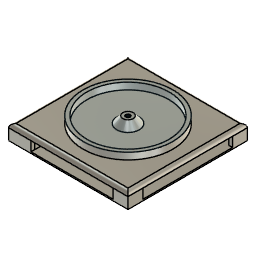
LED Box Holder (Autodesk Fusion 360 design; units mm, degrees)
Autodesk Fusion 360 part; units mm, degrees
sketch "Sketch1" plane through (0, 0, 0) normal (1, 0, 0) x (0, 1, 0)
  line L0 (-80, 80) -> (80, 80)
  line L1 (80, 80) -> (80, -80)
  line L2 (80, -80) -> (-80, -80)
  line L3 (-80, -80) -> (-80, 80)
  line L4 (-80, 80) -> (80, -80) construction
  line L5 (80, 80) -> (-80, -80) construction
  dimension "d1" = 160
  dimension "d2" = 160
  constraint horizontal L0
  constraint perpendicular L0 L1
  constraint parallel L0 L2
  constraint parallel L1 L3
  constraint coincident L4 origin
  constraint coincident L5 origin
  measures "d1" distance of L1.end L2.end
  measures "d2" distance of L0.end L1.end
extrude "Extrude1" add sketch "Sketch1" along normal blind 5 makes body 1
sketch "Sketch2" plane through (5, 0, 0) normal (1, 0, 0) x (0, 1, 0)
  line L0 (-80, -80) -> (80, -80)
  line L1 (80, -80) -> (80, 80)
  line L2 (80, 80) -> (-80, 80)
  line L3 (-80, 80) -> (-80, -80)
  line L4 (-55, 50) -> (55, 50)
  line L5 (55, 50) -> (55, 35)
  line L6 (55, 35) -> (-55, 35)
  line L7 (-55, 35) -> (-55, 50)
  dimension "d5" = 110
  dimension "d6" = 15
  dimension "d7" = 30
  dimension "d8" = 25
  constraint horizontal L4
  constraint vertical L5
  constraint horizontal L6
  constraint vertical L7
  measures "d5" distance of L4.start L4.end
  measures "d6" distance of L4.start L6.end
  measures "d7" distance of L2 L4
  measures "d8" distance of L1 L5
extrude "Extrude2" cut sketch "Sketch2" against normal blind 20 contours L4 L5 L6 L7 bodies 1
sketch "Sketch3" plane through (0, 0, 0) normal (-1, 0, 0) x (0, -1, 0)
  line L0 (-55, 35) -> (-55, 50)
  line L1 (-55, 50) -> (55, 50)
  line L2 (55, 50) -> (55, 35)
  line L3 (55, 35) -> (-55, 35)
  line L4 (-80, -80) -> (80, -80)
  line L5 (80, -80) -> (80, 80)
  line L6 (80, 80) -> (-80, 80)
  line L7 (-80, 80) -> (-80, -80)
  line L8 (-50, 35) -> (-30, 35)
  line L9 (-30, 35) -> (-30, -80)
  line L10 (-30, -80) -> (-50, -80)
  line L11 (-50, -80) -> (-50, 35)
  line L12 (-10, 35) -> (10, 35)
  line L13 (10, 35) -> (10, -80)
  line L14 (10, -80) -> (-10, -80)
  line L15 (-10, -80) -> (-10, 35)
  line L16 (30, 35) -> (50, 35)
  line L17 (50, 35) -> (50, -80)
  line L18 (50, -80) -> (30, -80)
  line L19 (30, -80) -> (30, 35)
  dimension "d11" = 20
  dimension "d12" = 115
  dimension "d13" = 20
  dimension "d14" = 115
  dimension "d15" = 5
  dimension "d17" = 20
  dimension "d18" = 20
  dimension "d19" = 115
  constraint horizontal L8
  constraint vertical L9
  constraint horizontal L10
  constraint vertical L11
  constraint coincident L3 L8.start
  constraint horizontal L12
  constraint vertical L13
  constraint horizontal L14
  constraint vertical L15
  constraint coincident L3 L12.start
  constraint horizontal L16
  constraint vertical L17
  constraint horizontal L18
  constraint vertical L19
  constraint coincident L3 L16.start
  measures "d11" distance of L8.start L8.end
  measures "d12" distance of L8.start L10.end
  measures "d13" distance of L12.start L12.end
  measures "d14" distance of L12.start L14.end
  measures "d15" distance of L0 L11
  measures "d17" distance of L9 L15
  measures "d18" distance of L13 L19
  measures "d19" distance of L16 L18
extrude "Extrude3" cut sketch "Sketch3" against normal blind 3 contours L3 L4 L8 L9 L10 L11 | L3 L4 L12 L13 L14 L15 | L3 L4 L16 L17 L18 L19 bodies 1
extrude "Extrude4" add 3 faces at (0, 18.3333, 70) (0, 23.3333, -41.6667) (0, -23.3333, -3.3333) along direction (-1, 0, 0) blind 10 on bodies 1 bodies 1
sketch "Sketch4" plane through (-10, 0, 0) normal (-1, 0, 0) x (0, -1, 0)
  line L0 (-50, -80) -> (-50, 35)
  line L1 (-50, 35) -> (-55, 35)
  line L2 (-55, 35) -> (-55, 50)
  line L3 (-55, 50) -> (55, 50)
  line L4 (55, 50) -> (55, 35)
  line L5 (55, 35) -> (50, 35)
  line L6 (50, 35) -> (50, -80)
  line L7 (50, -80) -> (80, -80)
  line L8 (80, -80) -> (80, 80)
  line L9 (80, 80) -> (-80, 80)
  line L10 (-80, 80) -> (-80, -80)
  line L11 (-80, -80) -> (-50, -80)
  line L12 (-80, -80) -> (80, -80)
  line L13 (80, -80) -> (80, 80)
  line L14 (80, 80) -> (-80, 80)
  line L15 (-80, 80) -> (-80, -80)
  dimension "d24" = 160
  constraint horizontal L12
  constraint vertical L13
  constraint horizontal L14
  constraint vertical L15
  constraint coincident L10.end L11.start
  measures "d24" distance of L10.end L9.end
extrude "Extrude5" add sketch "Sketch4" along normal blind 5 bodies 1
fillet "Fillet1" radius 5 4 edges at (-15, 0, 80) (-15, 80, 0) (-15, -80, 0) (-15, 0, -80) on bodies 1
sketch "Sketch5" plane through (-15, 0, 0) normal (-1, 0, 0) x (0, -1, 0)
  line L0 (-75, -75) -> (75, -75)
  line L1 (75, -75) -> (75, 75)
  line L2 (75, 75) -> (-75, 75)
  line L3 (-75, 75) -> (-75, -75)
  circle A0 centre (0, 0) radius 60
  constraint coincident A0.centre origin
extrude "Extrude6" add sketch "Sketch5" along normal blind 9 contours A0 bodies 1
sketch "Sketch6" plane through (-24, 0, 0) normal (-1, 0, 0) x (0, -1, 0)
  circle A0 centre (0, 0) radius 60
  circle A1 centre (0, 0) radius 3
  dimension "d31" = 6
  constraint coincident A0.centre A1.centre
  measures "d31" diameter of A1
extrude "Extrude7" cut sketch "Sketch6" against normal blind 10 contours A1 bodies 1
thread "Thread1" "ISO Metric profile 6.0 M6x1 6H" major diameter 6.147 minor diameter 5.035 pitch 1 angle 60 modelled right hand crest width 0.2748 on face at (-17.3333, -2.9963, -0.1495) crest through (-23.75, -2.5175, 0) on bodies 1
sketch "Sketch7" plane through (-24, 0, 0) normal (-1, 0, 0) x (0, -1, 0)
  spline S0 degree 3 poles (-0.7938, -2.9692) (-1.1619, -2.8346) (-1.5007, -2.6305) (-2.069, -2.1114) (-2.2965, -1.8052) (-2.6132, -1.1343) (-2.704, -0.7783) (-2.7408, -0.0652) (-2.6916, 0.2847) (-2.5067, 0.8107) (-2.4149, 0.9977) (-2.1912, 1.3413) (-2.061, 1.4974) (-1.9135, 1.636) knots 0 0 0 0 0.117588 0.117588 0.231087 0.231087 0.340498 0.340498 0.445817 0.445817 0.508297 0.508297 0.569249 0.569249 0.569249 0.569249
  arc A0 (1.9135, 1.636) -> (-1.9135, 1.636) centre (0, 0) ccw
  spline S1 degree 3 poles (1.9135, 1.636) (2.1558, 1.4082) (2.3504, 1.1345) (2.6319, 0.5162) (2.7113, 0.1755) (2.7381, -0.5311) (2.68, -0.8904) (2.4271, -1.5805) (2.2298, -1.9028) (1.817, -2.3542) (1.6364, -2.5092) (1.2382, -2.776) (1.0214, -2.886) (0.7938, -2.9692) knots 0 0 0 0 0.09977 0.09977 0.203618 0.203618 0.311544 0.311544 0.423544 0.423544 0.494428 0.494428 0.566847 0.566847 0.566847 0.566847
  arc A1 (-0.7938, -2.9692) -> (0.7938, -2.9692) centre (0, 0) ccw
  circle A2 centre (0, 0) radius 60
  circle A3 centre (0, 0) radius 55
  circle A4 centre (0, 0) radius 15
  constraint coincident A0.centre A1.centre
  constraint concentric A3 A4
extrude "Extrude8" cut sketch "Sketch7" against normal blind 9 contours A3 bodies 1
chamfer "Chamfer1" distance 8 distance2 9 1 edges at (-24, 13.9849, -5.4242) measured on face at (-24, 0, 10.8112) on bodies 1
copy_body "Body->Comp1" bodies 1 removing the originals makes body 2 in component "Component"
move_body "Move1" bodies 2 to x (0, 0, -1) y (0, -1, 0) z (-1, 0, 0) at (5, 0, 5) in component "Component"
sketch "Sketch8" plane through (85, 0, 0) normal (1, 0, 0) x (0, 1, 0)
  line L0 (-50, 15) -> (-80, 15)
  line L1 (-80, 15) -> (-80, 0)
  line L2 (-80, 0) -> (80, 0)
  line L3 (80, 0) -> (80, 15)
  line L4 (80, 15) -> (50, 15)
  line L5 (50, 15) -> (50, 2)
  line L6 (50, 2) -> (30, 2)
  line L7 (30, 2) -> (30, 15)
  line L8 (30, 15) -> (10, 15)
  line L9 (10, 15) -> (10, 2)
  line L10 (10, 2) -> (-10, 2)
  line L11 (-10, 2) -> (-10, 15)
  line L12 (-10, 15) -> (-30, 15)
  line L13 (-30, 15) -> (-30, 2)
  line L14 (-30, 2) -> (-50, 2)
  line L15 (-50, 2) -> (-50, 15)
  line L16 (-75, 15) -> (75, 15)
  line L17 (75, 15) -> (75, 2)
  line L18 (75, 2) -> (-75, 2)
  line L19 (-75, 2) -> (-75, 15)
  dimension "d40" = 150
  constraint horizontal L16
  constraint vertical L17
  constraint horizontal L18
  constraint vertical L19
  constraint coincident L0 L16.start
  measures "d40" distance of L16.start L16.end
extrude "Extrude1'" cut sketch "Sketch8" against normal blind 130 contours L0 L15 L16 L18 L19 | L4 L5 L16 L17 L18 bodies 2 in component "Component"
sketch "Sketch9" plane through (85, 0, 0) normal (1, 0, 0) x (0, 1, 0)
  line L0 (-75, 2) -> (-75, 15)
  line L1 (-75, 15) -> (-80, 15)
  line L2 (-80, 15) -> (-80, 0)
  line L3 (-80, 0) -> (80, 0)
  line L4 (80, 0) -> (80, 15)
  line L5 (80, 15) -> (75, 15)
  line L6 (75, 15) -> (75, 2)
  line L7 (75, 2) -> (30, 2)
  line L8 (30, 2) -> (30, 15)
  line L9 (30, 15) -> (10, 15)
  line L10 (10, 15) -> (10, 2)
  line L11 (10, 2) -> (-10, 2)
  line L12 (-10, 2) -> (-10, 15)
  line L13 (-10, 15) -> (-30, 15)
  line L14 (-30, 15) -> (-30, 2)
  line L15 (-30, 2) -> (-75, 2)
  line L16 (-10, 15) -> (-15, 15)
  line L17 (-15, 15) -> (-15, 2)
  line L18 (-15, 2) -> (-10, 2)
  line L19 (-10, 2) -> (-10, 15)
  line L20 (10, 15) -> (15, 15)
  line L21 (15, 15) -> (15, 2)
  line L22 (15, 2) -> (10, 2)
  line L23 (10, 2) -> (10, 15)
  dimension "d43" = 5
  dimension "d44" = 13
  dimension "d45" = 5
  dimension "d46" = 13
  constraint horizontal L16
  constraint vertical L17
  constraint horizontal L18
  constraint vertical L19
  constraint coincident L12.end L13.start
  constraint horizontal L20
  constraint vertical L21
  constraint horizontal L22
  constraint vertical L23
  constraint coincident L9.end L10.start
  measures "d43" distance of L12.end L16.end
  measures "d44" distance of L12.end L11.end
  measures "d45" distance of L9.end L20.end
  measures "d46" distance of L9.end L10.end
extrude "Extrude2'" cut sketch "Sketch9" against normal blind 120 contours L12 L13 L16 L17 L18 L19 | L9 L10 L20 L21 L22 L23 bodies 2 in component "Component"
sketch "Sketch10" plane through (0, 80, 0) normal (0, 1, 0) x (-1, 0, 0)
  line L0 (75, 15) -> (-85, 15)
  line L1 (-85, 15) -> (-85, 0)
  line L2 (-85, 0) -> (75, 0)
  line L3 (75, 0) -> (75, 15)
  line L4 (-65, 15) -> (55, 15)
  line L5 (55, 15) -> (55, 3)
  line L6 (55, 3) -> (-65, 3)
  line L7 (-65, 3) -> (-65, 15)
  dimension "d49" = 120
  dimension "d50" = 12
  constraint horizontal L4
  constraint vertical L5
  constraint horizontal L6
  constraint vertical L7
  constraint coincident L0 L4.start
  measures "d49" distance of L4.start L4.end
  measures "d50" distance of L4.start L6.end
extrude "Extrude3'" cut sketch "Sketch10" against normal blind 8 contours L0 L4 L5 L6 L7 bodies 2 in component "Component"
extrude "Extrude4'" add 1 faces at (-48.3333, 72, 11) along direction (0, 1, 0) blind 8 on bodies 2 bodies 2 in component "Component"
sketch "Sketch11" plane through (0, -80, 0) normal (0, -1, 0) x (1, 0, 0)
  line L0 (85, 15) -> (-75, 15)
  line L1 (-75, 15) -> (-75, 0)
  line L2 (-75, 0) -> (85, 0)
  line L3 (85, 0) -> (85, 15)
  line L4 (-55, 15) -> (65, 15)
  line L5 (65, 15) -> (65, 3)
  line L6 (65, 3) -> (-55, 3)
  line L7 (-55, 3) -> (-55, 15)
  dimension "d55" = 120
  dimension "d56" = 12
  constraint horizontal L4
  constraint vertical L5
  constraint horizontal L6
  constraint vertical L7
  constraint coincident L0 L4.start
  measures "d55" distance of L4.start L4.end
  measures "d56" distance of L4.start L6.end
extrude "Extrude5'" cut sketch "Sketch11" against normal blind 5 contours L0 L4 L5 L6 L7 bodies 2 in component "Component"
extrude "Extrude6'" add 1 faces at (-48.3333, -75, 11) along direction (0, -1, 0) blind 5 on bodies 2 bodies 2 in component "Component"
extrude "Extrude7'" cut 1 faces at (28.3333, -78.3333, 3) along direction (0, 0, -1) blind 1 on bodies 2 bodies 2 in component "Component"
extrude "Extrude8'" cut 1 faces at (-8.3333, 78.3333, 3) along direction (0, 0, -1) blind 1 on bodies 2 bodies 2 in component "Component"
sketch "Sketch12" plane through (85, 0, 0) normal (1, 0, 0) x (0, 1, 0)
  line L0 (15, 2) -> (-15, 2)
  line L1 (-15, 2) -> (-15, 15)
  line L2 (-15, 15) -> (-30, 15)
  line L3 (-30, 15) -> (-30, 2)
  line L4 (-30, 2) -> (-75, 2)
  line L5 (-75, 2) -> (-75, 15)
  line L6 (-75, 15) -> (-80, 15)
  line L7 (-80, 15) -> (-80, 0)
  line L8 (-80, 0) -> (80, 0)
  line L9 (80, 0) -> (80, 15)
  line L10 (80, 15) -> (75, 15)
  line L11 (75, 15) -> (75, 2)
  line L12 (75, 2) -> (30, 2)
  line L13 (30, 2) -> (30, 15)
  line L14 (30, 15) -> (15, 15)
  line L15 (15, 15) -> (15, 2)
  line L16 (-30, 15) -> (30, 15)
  line L17 (30, 15) -> (30, 2)
  line L18 (30, 2) -> (-30, 2)
  line L19 (-30, 2) -> (-30, 15)
  constraint horizontal L16
  constraint vertical L17
  constraint horizontal L18
  constraint vertical L19
  constraint coincident L12.end L13.start
  constraint coincident L2.end L3.start
extrude "Extrude9" cut sketch "Sketch12" against normal blind 115 contours L13 L14 L15 L16 L17 L18 | L1 L2 L3 L16 L18 L19 bodies 2 in component "Component"
sketch "Sketch13" plane through (0, -75, 0) normal (0, 1, 0) x (-1, 0, 0)
  line L0 (-65, 2) -> (-65, 15)
  line L1 (-65, 15) -> (-85, 15)
  line L2 (-85, 15) -> (-85, 2)
  line L3 (-85, 2) -> (-65, 2)
  line L4 (-85, 15) -> (-80, 15)
  line L5 (-80, 15) -> (-80, 2)
  line L6 (-80, 2) -> (-85, 2)
  line L7 (-85, 2) -> (-85, 15)
  dimension "d67" = 5
  constraint horizontal L4
  constraint vertical L5
  constraint horizontal L6
  constraint vertical L7
  constraint coincident L1.end L2.start
  measures "d67" distance of L1.end L4.end
extrude "Extrude10" add sketch "Sketch13" along normal blind 15 contours L1 L2 L3 L4 L5 L6 L7 bodies 2 in component "Component"
sketch "Sketch14" plane through (0, 75, 0) normal (0, -1, 0) x (1, 0, 0)
  line L0 (65, 15) -> (65, 2)
  line L1 (65, 2) -> (85, 2)
  line L2 (85, 2) -> (85, 15)
  line L3 (85, 15) -> (65, 15)
  line L4 (85, 15) -> (80, 15)
  line L5 (80, 15) -> (80, 2)
  line L6 (80, 2) -> (85, 2)
  line L7 (85, 2) -> (85, 15)
  dimension "d70" = 5
  constraint horizontal L4
  constraint vertical L5
  constraint horizontal L6
  constraint vertical L7
  constraint coincident L2.end L3.start
  measures "d70" distance of L2.end L4.end
extrude "Extrude11" add sketch "Sketch14" along normal blind 15 contours L1 L2 L3 L4 L5 L6 L7 bodies 2 in component "Component"
sketch "Sketch15" plane through (-45, 0, 0) normal (1, 0, 0) x (0, 1, 0)
  line L0 (80, 2) -> (80, 15)
  line L1 (80, 15) -> (-80, 15)
  line L2 (-80, 15) -> (-80, 2)
  line L3 (-80, 2) -> (-55, 2)
  line L4 (-55, 2) -> (-55, 0)
  line L5 (-55, 0) -> (55, 0)
  line L6 (55, 0) -> (55, 2)
  line L7 (55, 2) -> (80, 2)
  line L8 (-60, 2) -> (60, 2)
  line L9 (60, 2) -> (60, 15)
  line L10 (60, 15) -> (-60, 15)
  line L11 (-60, 15) -> (-60, 2)
  constraint horizontal L8
  constraint vertical L9
  constraint horizontal L10
  constraint vertical L11
  constraint coincident L1 L9.end
  constraint coincident L3 L8.start
extrude "Extrude12" cut sketch "Sketch15" against normal blind 25 contours L1 L3 L7 L8 L9 L10 L11 bodies 2 in component "Component"
sketch "Sketch16" plane through (-45, 0, 0) normal (1, 0, 0) x (0, 1, 0)
  line L0 (-60, 2) -> (-60, 15)
  line L1 (-60, 15) -> (-80, 15)
  line L2 (-80, 15) -> (-80, 2)
  line L3 (-80, 2) -> (-60, 2)
  line L4 (-80, 15) -> (-75, 15)
  line L5 (-75, 15) -> (-75, 2)
  line L6 (-75, 2) -> (-80, 2)
  line L7 (-80, 2) -> (-80, 15)
  constraint horizontal L4
  constraint vertical L5
  constraint horizontal L6
  constraint vertical L7
  constraint coincident L3 L5.end
  constraint coincident L1.end L2.start
extrude "Extrude13" cut sketch "Sketch16" against normal blind 25 contours L0 L1 L3 L5 bodies 2 in component "Component"
sketch "Sketch17" plane through (-45, 0, 0) normal (1, 0, 0) x (0, 1, 0)
  line L0 (60, 15) -> (60, 2)
  line L1 (60, 2) -> (80, 2)
  line L2 (80, 2) -> (80, 15)
  line L3 (80, 15) -> (60, 15)
  line L4 (80, 15) -> (75, 15)
  line L5 (75, 15) -> (75, 2)
  line L6 (75, 2) -> (80, 2)
  line L7 (80, 2) -> (80, 15)
  constraint horizontal L4
  constraint vertical L5
  constraint horizontal L6
  constraint vertical L7
  constraint coincident L1 L5.end
  constraint coincident L2.end L3.start
extrude "Extrude14" cut sketch "Sketch17" against normal blind 25 contours L0 L1 L3 L5 bodies 2 in component "Component"
sketch "Sketch18" plane through (0, 0, 29) normal (0, 0, 1) x (-1, 0, 0)
  circle A0 centre (-5, 0) radius 60
  circle A1 centre (-5, 0) radius 55
component "Component" placed x (1, 0, 0) y (0, 1, 0) z (0, 0, 1) at (0, 0, 0)
